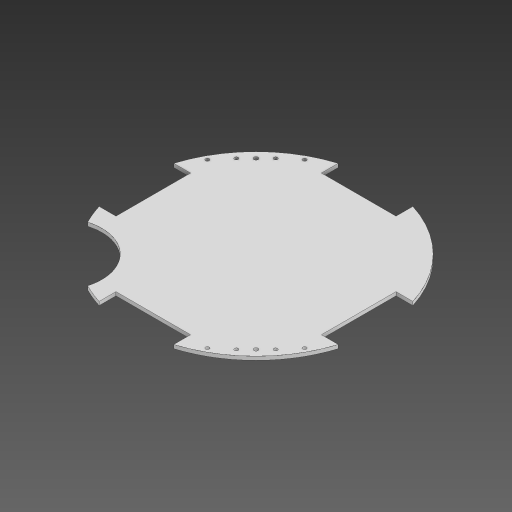
# Autodesk Inventor part: top
Saved by Autodesk Inventor 2023 (Build 270158000, 158)
## iProperties
Created: 2025-06-24
Part Number: top
Material: Типовые
Document SubType Name: Modeling
Designer: daa
Density: 1 g/cm^3
Appearance: По умолчанию
Author: daa
Autodesk Inventor part; units mm, degrees
ref_plane "YZ Plane" through (0, 0, 0) normal (1, 0, 0) x (0, 1, 0)
ref_plane "XZ Plane" through (0, 0, 0) normal (0, 1, 0) x (-1, 0, 0)
ref_plane "XY Plane" through (0, 0, 0) normal (0, 0, 1) x (1, 0, 0)
sketch "Эскиз1" plane through (0, 0, 0) normal (0, 1, 0) x (-1, 0, 0)
  line L0 (-79, -47.2724) -> (-79, 14.7276)
  line L1 (91.5447, -47.2724) -> (91.5447, 14.7276)
  line L2 (-79, -47.2724) -> (-93, -47.2724)
  line L3 (-79, 14.7276) -> (-93, 14.7276)
  line L4 (91.5447, -47.2724) -> (105.5447, -47.2724)
  line L5 (91.5447, 14.7276) -> (105.5447, 14.7276)
  line L6 (-24.7276, -101.5447) -> (37.2724, -101.5447)
  line L7 (-24.7276, 69) -> (37.2724, 69)
  line L8 (-24.7276, 69) -> (-24.7276, 83)
  line L9 (37.2724, 69) -> (37.2724, 83)
  line L10 (37.2724, -101.5447) -> (37.2724, -115.5447)
  line L11 (-24.7276, -101.5447) -> (-24.7276, -115.5447)
  arc A0 (-93, -47.2724) -> (-24.7276, -115.5447) centre (6.2724, -16.2724) ccw
  arc A1 (105.5447, 14.7276) -> (37.2724, 83) centre (6.2724, -16.2724) ccw
  arc A2 (-24.7276, 83) -> (-93, 14.7276) centre (6.2724, -16.2724) ccw
  arc A3 (37.2724, -115.5447) -> (105.5447, -47.2724) centre (6.2724, -16.2724) ccw
  dimension "d29" = 62
  dimension "d31" = 62
  dimension "d33" = 14
  dimension "d34" = 14
  dimension "d35" = 62
  dimension "d36" = 62
  dimension "d39" = 14
  dimension "d40" = 14
  constraints: 24 end point, 8 point on circle, 4 centre point, 4 horizontal, 3 parallel, 3 vertical, 2 point on line, 1 concentric
  measures "d29" distance of L0.start L0.end
  measures "d31" distance of L1.start L1.end
  measures "d33" distance of L0.end L3.end
  measures "d34" distance of L1.end L5.end
  measures "d35" distance of L6.start L6.end
  measures "d36" distance of L7.start L7.end
  measures "d39" distance of L7.start L8.end
  measures "d40" distance of L6.start L11.end
extrude "Выдавливание1" add sketch "Эскиз1" along normal blind 3
sketch "Эскиз2" plane through (0, 3, 0) normal (0, 1, 0) x (1, 0, 0)
  line L0 (-37.2724, -83) -> (-37.2724, -69) projected
  line L1 (-91.5447, -14.7276) -> (-105.5447, -14.7276) projected
  line L2 (-37.2724, -69) -> (-91.5447, -14.7276)
  line L3 (-37.2724, -69) -> (-41.515, -64.7574)
  line L4 (-91.5447, -14.7276) -> (-87.3021, -18.9703)
  line L5 (-41.515, -64.7574) -> (-53.253, -76.4953)
  line L6 (-87.3021, -18.9703) -> (-99.04, -30.7083)
  arc A0 (-53.253, -76.4953) -> (-99.04, -30.7083) centre (-88.8109, -66.2662) ccw
  arc A1 (-53.253, -76.4953) -> (-37.2724, -83) centre (-6.1897, 16.2465) ccw
  arc A2 (-105.5447, -14.7276) -> (-37.2724, -83) centre (-6.2724, 16.2724) ccw projected
  arc A3 (-105.5447, -14.7276) -> (-99.04, -30.7083) centre (-6.2982, 16.355) ccw
  point P0 (0, 0)
  dimension "d47" = 6
  dimension "d48" = 6
  dimension "d49" = 16.6
  dimension "d50" = 16.6
  dimension "d51" = 37
  dimension "d52" = 104
  dimension "d53" = 104
  dimension "d54" = 6.5047
  constraints: 10 end point, 6 point on circle, 3 centre point, 2 point on line, 1 perpendicular
  measures "d47" distance of L0.end L3.end
  measures "d48" distance of L1.start L4.end
  measures "d49" distance of L3.end L5.end
  measures "d50" distance of L4.end L6.end
  measures "d51" radius of A0
  measures "d52" radius of A1
  measures "d53" radius of A3
  measures "d54" vertical distance of L5.end L0.start
extrude "Выдавливание2" cut sketch "Эскиз2" against normal blind 3 contours A2 A3 A0 L2 A1 | L2 A0
sketch "Эскиз3" plane through (0, 3, 0) normal (0, 1, 0) x (1, 0, 0)
  arc A0 (93, 47.2724) -> (24.7276, 115.5447) centre (-6.2724, 16.2724) ccw projected
  line L0 (-6.2724, 16.2724) -> (97.7276, 16.2724) construction
  line L1 (67.2668, 89.8115) -> (-62.5447, -40)
  circle A1 centre (62.3989, -52.3991) radius 1.75
  circle A2 centre (70.5306, -44.2673) radius 1.5
  circle A3 centre (54.2672, -60.5308) radius 1.5
  circle A4 centre (41.3053, -71.6104) radius 1.5
  circle A5 centre (81.6104, -31.3053) radius 1.5
  arc A6 (24.7276, -83) -> (93, -14.7276) centre (-6.2724, 16.2724) ccw projected
  line L2 (-6.2724, 16.2724) -> (97.7276, 16.2724) construction
  line L3 (-79.8115, 89.8115) -> (67.2668, -57.2668)
  line L4 (-91.5447, 47.2724) -> (-91.5447, -14.7276) projected
  line L5 (-91.5447, 16.2724) -> (79, 16.2724)
  line L6 (24.7276, 101.5447) -> (-37.2724, 101.5447) projected
  line L7 (-6.2724, 101.5447) -> (-6.2724, -69)
  line L8 (-6.2724, 101.5447) -> (-6.2724, -69)
  line L9 (-91.5447, 47.2724) -> (-91.5447, -14.7276) projected
  arc A7 (24.7276, -83) -> (93, -14.7276) centre (-6.2724, 16.2724) ccw projected
  circle A8 centre (-74.9438, 84.9436) radius 1.75
  circle A9 centre (-66.812, 93.0753) radius 1.5
  circle A10 centre (-83.0755, 76.8119) radius 1.5
  circle A11 centre (-94.1551, 63.85) radius 1.5
  circle A12 centre (-53.85, 104.1551) radius 1.5
  point P0 (0, 0)
  point P1 (67.2668, -57.2668)
  point P2 (67.2668, -57.2668)
  point P3 (-105.5447, 47.2724)
  point P4 (-79.8115, 89.8115)
  point P5 (-79.8115, 89.8115)
  point P6 (-79.8115, 89.8115)
  dimension "d64" = 3.5
  dimension "d65" = 3
  dimension "d66" = 3
  dimension "d67" = 3
  dimension "d68" = 3
  dimension "d69" = 23
  dimension "d70" = 11.5
  dimension "d71" = 57
  dimension "d74" = -12.962
  dimension "d77" = 4.8677
  dimension "d78" = 25.9614
  constraints: 14 end point, 10 centre point, 9 symmetric about line, 4 point on circle, 3 midpoint, 2 horizontal, 2 vertical, 1 point on line, 5 other
  measures "d64" diameter of A1
  measures "d65" diameter of A2
  measures "d66" diameter of A3
  measures "d67" diameter of A4
  measures "d68" diameter of A5
  measures "d69" distance of A3.centre A2.centre
  measures "d70" distance of A3.centre A1.centre
  measures "d71" distance of A4.centre A5.centre
  measures "d74" vertical distance of A2.centre A5.centre
  measures "d77" vertical distance of point (67.267, -57.267) A1.centre
  measures "d78" vertical distance of A5.centre point (67.267, -57.267)
extrude "Выдавливание3" cut sketch "Эскиз3" against normal blind 10
